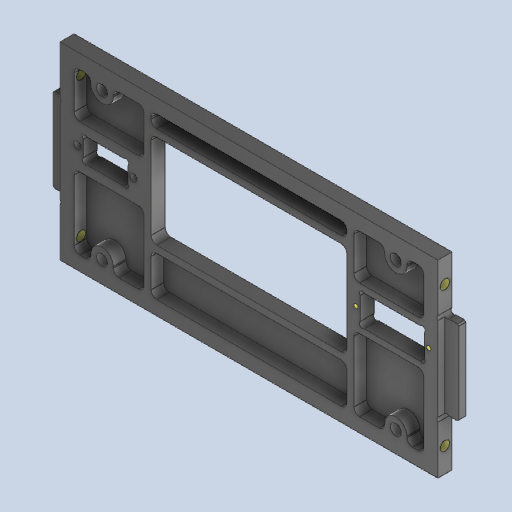
# Autodesk Inventor part: Cockpit_back_frame
Saved by Autodesk Inventor 2022.3 (Build 263350000, 350)
## iProperties
Part Number: Cockpit_back_frame
Material: アセタール樹脂、黒
Document SubType Name: Modeling
Designer: Masato Kubotera
Density: 1.425 g/cm^3
Appearance: 滑らか - 黒
Description: POM T5
Mass: 27.6157 g
Surface Area: 210.6 cm^2
Volume: 19.3794 cm^3
Author: Masato Kubotera
Autodesk Inventor part; units mm, degrees
ref_plane "XZ Plane" through (0, 0, 0) normal (0, 1, 0) x (-1, 0, 0)
derived "Cockpit_side_frame.ipt"
sketch "スケッチ2" plane through (0, 0, 0) normal (0, 1, 0) x (-1, 0, 0)
  line L0 (-23.5, -22.5) -> (-28.5, -27.5)
  line L1 (-28.5, -27.5) -> (-28.5, -91)
  line L2 (-28.5, -91) -> (-23.5, -96)
  line L3 (-23.5, -96) -> (34.25, -96)
  line L4 (36.25, -98) -> (36.25, -128.5)
  line L5 (36.25, -128.5) -> (46.25, -138.5)
  line L6 (46.25, -138.5) -> (86.5, -138.5)
  line L7 (91.5, -133.5) -> (91.5, -20)
  line L8 (91.5, -20) -> (89, -17.5)
  line L9 (89, -17.5) -> (83.25, -17.5)
  line L10 (83.25, -17.5) -> (83.25, -21.0151)
  line L11 (81.7651, -22.5) -> (76.8599, -22.5)
  line L12 (75.375, -21.0151) -> (75.375, -17.5)
  line L13 (75.375, -17.5) -> (60.375, -17.5)
  line L14 (60.375, -17.5) -> (60.375, -21.0151)
  line L15 (58.8901, -22.5) -> (-23.5, -22.5)
  line L16 (-25.25, -25) -> (-20.25, -25) construction
  line L17 (-20.25, -25) -> (-20.25, -93.5) construction
  line L18 (-20.25, -93.5) -> (-25.25, -93.5) construction
  line L19 (-25.25, -93.5) -> (-25.25, -25) construction
  line L20 (-26, -25) -> (-25.25, -25) construction
  line L21 (-25.25, -93.5) -> (-26, -93.5) construction
  line L22 (-26, -93.5) -> (-26, -25) construction
  line L23 (-20.25, -93.5) -> (83.25, -93.5) construction
  line L24 (-20.25, -88.5) -> (83.25, -88.5) construction
  line L25 (83.25, -22.5) -> (83.25, -90) construction
  line L26 (83.25, -90) -> (88.25, -90) construction
  line L27 (88.25, -90) -> (88.25, -22.5) construction
  line L28 (83.25, -88.5) -> (83.25, -93.5) construction
  line L29 (83.25, -91) -> (88.25, -91) construction
  line L30 (88.25, -91) -> (88.25, -136) construction
  line L31 (83.25, -91) -> (83.25, -136) construction
  line L32 (83.25, -136) -> (88.25, -136) construction
  line L33 (38.75, -131) -> (38.75, -93.5) construction
  line L34 (43.75, -93.5) -> (43.75, -131) construction
  line L35 (38.75, -131) -> (43.75, -131) construction
  line L36 (41.25, -131) -> (41.25, -93.5) construction
  line L37 (43.75, -131) -> (81.25, -131) construction
  line L38 (81.25, -131) -> (81.25, -136) construction
  line L39 (81.25, -136) -> (43.75, -136) construction
  line L40 (43.75, -133.5) -> (81.25, -133.5) construction
  line L41 (85.75, -91) -> (85.75, -136) construction
  circle A0 centre (85.75, -133.5) radius 2.975
  arc A1 (83.25, -131) -> (88.25, -131) centre (85.75, -133.5) ccw construction
  line L42 (83.25, -91) -> (-20.25, -91) construction
  line L43 (41.25, -112.25) -> (43.75, -112.25) construction
  line L44 (62.5, -131) -> (62.5, -133.5) construction
  line L45 (41.2, -116.8151) -> (41.2, -107.6849)
  line L46 (43.8, -108.3) -> (43.8, -116.2)
  line L47 (43.8, -118.3) -> (41.2, -106.2) construction
  line L48 (41.2, -118.3) -> (43.8, -106.2) construction
  line L49 (58.55, -130.95) -> (66.45, -130.95)
  line L50 (67.0651, -133.55) -> (57.9349, -133.55)
  line L51 (56.45, -130.95) -> (68.55, -133.55) construction
  line L52 (68.55, -130.95) -> (56.45, -133.55) construction
  line L53 (41.25, -106.25) -> (43.75, -106.25) construction
  line L54 (41.25, -118.25) -> (43.75, -118.25) construction
  arc A2 (42.6849, -106.2) -> (41.2, -107.6849) centre (41.9425, -106.9425) ccw
  arc A3 (43.8, -108.3) -> (43.8, -106.2) centre (43.8, -107.25) ccw
  arc A4 (41.2, -116.8151) -> (42.6849, -118.3) centre (41.9425, -117.5575) ccw
  arc A5 (43.8, -118.3) -> (43.8, -116.2) centre (43.8, -117.25) ccw
  line L55 (56.5, -133.5) -> (56.5, -131) construction
  line L56 (68.5, -131) -> (68.5, -133.5) construction
  arc A6 (56.45, -132.0651) -> (57.9349, -133.55) centre (57.1925, -132.8075) ccw
  arc A7 (58.55, -130.95) -> (56.45, -130.95) centre (57.5, -130.95) ccw
  arc A8 (67.0651, -133.55) -> (68.55, -132.0651) centre (67.8075, -132.8075) ccw
  arc A9 (68.55, -130.95) -> (66.45, -130.95) centre (67.5, -130.95) ccw
  line L57 (56.45, -132.0651) -> (56.45, -130.95)
  line L58 (68.55, -130.95) -> (68.55, -132.0651)
  line L59 (42.6849, -106.2) -> (43.8, -106.2)
  line L60 (43.8, -118.3) -> (42.6849, -118.3)
  circle A10 centre (48.75, -133.5) radius 1.6
  line L61 (88.25, -22.5) -> (88.25, -17.5) construction
  line L62 (89, -17.5) -> (89, -90) construction
  line L63 (89, -90) -> (88.25, -90) construction
  line L64 (-13.5, -82.5) -> (-13.5, -61)
  arc A11 (-13.5, -82.5) -> (-11.5, -84.5) centre (-11.5, -82.5) ccw
  line L65 (45.5, -84.5) -> (-11.5, -84.5)
  arc A12 (45.5, -84.5) -> (47.5, -82.5) centre (45.5, -82.5) ccw
  line L66 (47.5, -61) -> (47.5, -82.5)
  arc A13 (47.5, -61) -> (45.5, -59) centre (45.5, -61) ccw
  line L67 (-11.5, -59) -> (45.5, -59)
  arc A14 (-11.5, -59) -> (-13.5, -61) centre (-11.5, -61) ccw
  line L68 (31.5, -88.5) -> (31.5, -91) construction
  line L69 (85.75, -22.5) -> (85.75, -90) construction
  circle A15 centre (85.75, -31.25) radius 1.6
  circle A16 centre (85.75, -31.25) radius 3
  circle A17 centre (85.75, -81.25) radius 3
  circle A18 centre (85.75, -81.25) radius 1.6
  line L70 (88.25, -22.5) -> (83.25, -22.5) construction
  arc A19 (88.25, -91) -> (83.25, -91) centre (85.75, -133.5) ccw construction
  circle A20 centre (48.75, -133.5) radius 3
  circle A21 centre (41.25, -98.5) radius 1.6
  circle A22 centre (41.25, -98.5) radius 3
  line L71 (10.55, -88.5) -> (10.55, -91) construction
  line L72 (52.45, -88.5) -> (52.45, -91) construction
  line L73 (51.0151, -91.05) -> (11.9849, -91.05)
  line L74 (10.5, -89.5651) -> (10.5, -88.45)
  line L75 (12.6, -88.45) -> (50.4, -88.45)
  line L76 (52.5, -88.45) -> (52.5, -89.5651)
  line L77 (52.5, -91.05) -> (10.5, -88.45) construction
  line L78 (10.5, -91.05) -> (52.5, -88.45) construction
  arc A23 (12.6, -88.45) -> (10.5, -88.45) centre (11.55, -88.45) ccw
  arc A24 (10.5, -89.5651) -> (11.9849, -91.05) centre (11.2425, -90.3075) ccw
  arc A25 (51.0151, -91.05) -> (52.5, -89.5651) centre (51.7575, -90.3075) ccw
  arc A26 (52.5, -88.45) -> (50.4, -88.45) centre (51.45, -88.45) ccw
  line L79 (-20.25, -31) -> (83.25, -31) construction
  line L80 (83.25, -26) -> (-20.25, -26) construction
  line L81 (-20.25, -26) -> (-20.25, -31) construction
  line L82 (-20.25, -28.5) -> (83.25, -28.5) construction
  line L83 (31.5, -31) -> (31.5, -26) construction
  line L84 (11.9849, -31) -> (51.0151, -31)
  arc A27 (10.5, -29.5151) -> (11.9849, -31) centre (11.2425, -30.2575) ccw
  arc A28 (51.0151, -31) -> (52.5, -29.5151) centre (51.7575, -30.2575) ccw
  line L85 (10.55, -31) -> (10.55, -26) construction
  line L86 (52.45, -26) -> (52.45, -31) construction
  circle A29 centre (6.5, -28.5) radius 1.6
  circle A30 centre (6.5, -28.5) radius 3
  line L87 (-26, -59.25) -> (-25.25, -59.25) construction
  line L88 (-22.75, -25) -> (-22.75, -93.5) construction
  arc A31 (58.8901, -22.5) -> (60.375, -21.0151) centre (59.6325, -21.7575) ccw
  arc A32 (75.375, -21.0151) -> (76.8599, -22.5) centre (76.1175, -21.7575) ccw
  line L89 (56.4375, -22.5) -> (56.4375, -17.5) construction
  line L90 (79.3125, -22.5) -> (79.3125, -17.5) construction
  circle A33 centre (-22.75, -31.75) radius 1.6
  circle A34 centre (-22.75, -31.75) radius 3
  circle A35 centre (-22.75, -86.75) radius 1.6
  circle A36 centre (-22.75, -86.75) radius 3
  line L91 (60.375, -22.5) -> (75.375, -22.5)
  line L92 (52.5, -17.5) -> (52.5, -22.5) construction
  circle A37 centre (85.75, -98.5) radius 1.475
  circle A38 centre (85.75, -103.5) radius 1.475
  circle A39 centre (85.75, -108.5) radius 1.475
  line L93 (59.5, -88.5) -> (78.75, -88.5)
  line L94 (80.75, -90.5) -> (80.75, -126.5)
  line L95 (78.75, -128.5) -> (48.25, -128.5)
  line L96 (46.25, -126.5) -> (46.25, -110)
  arc A40 (46.25, -126.5) -> (48.25, -128.5) centre (48.25, -126.5) ccw
  arc A41 (78.75, -128.5) -> (80.75, -126.5) centre (78.75, -126.5) ccw
  arc A42 (80.75, -90.5) -> (78.75, -88.5) centre (78.75, -90.5) ccw
  arc A43 (36.25, -98) -> (34.25, -96) centre (34.25, -98) ccw
  circle A44 centre (-13.5, -55) radius 1.75
  circle A45 centre (-13.5, -55) radius 2
  line L97 (23.9, -43.85) -> (10.1, -43.85) construction
  line L98 (10.1, -43.85) -> (10.1, -34.65) construction
  line L99 (10.1, -34.65) -> (23.9, -34.65) construction
  line L100 (23.9, -34.65) -> (23.9, -43.85) construction
  line L101 (23.9, -43.85) -> (10.1, -34.65) construction
  line L102 (10.1, -43.85) -> (23.9, -34.65) construction
  line L103 (9.45, -33.95) -> (24.55, -33.95) construction
  line L104 (24.55, -33.95) -> (24.55, -44.55) construction
  line L105 (24.55, -44.55) -> (9.45, -44.55) construction
  line L106 (9.45, -44.55) -> (9.45, -33.95) construction
  line L107 (9.45, -33.95) -> (24.55, -44.55) construction
  line L108 (24.55, -33.95) -> (9.45, -44.55) construction
  line L109 (10.8849, -33.9) -> (23.1151, -33.9)
  line L110 (24.6, -35.3849) -> (24.6, -43.1151)
  line L111 (24.6, -44.6) -> (9.4, -33.9) construction
  line L112 (9.4, -44.6) -> (24.6, -33.9) construction
  line L113 (23.95, -43.9) -> (10.05, -34.6) construction
  line L114 (10.05, -43.9) -> (23.95, -34.6) construction
  arc A46 (10.8849, -33.9) -> (9.4, -35.3849) centre (10.1425, -34.6425) ccw
  arc A47 (11.5349, -34.6) -> (10.05, -36.0849) centre (10.7925, -35.3425) ccw
  line L115 (9.4, -39.25) -> (24.6, -39.25) construction
  line L116 (17, -33.9) -> (17, -44.6) construction
  arc A48 (24.6, -35.3849) -> (23.1151, -33.9) centre (23.8575, -34.6425) ccw
  arc A49 (23.95, -36.0849) -> (22.4651, -34.6) centre (23.2075, -35.3425) ccw
  arc A50 (10.05, -42.4151) -> (11.5349, -43.9) centre (10.7925, -43.1575) ccw
  arc A51 (9.4, -43.1151) -> (10.8849, -44.6) centre (10.1425, -43.8575) ccw
  arc A52 (22.4651, -43.9) -> (23.95, -42.4151) centre (23.2075, -43.1575) ccw
  arc A53 (23.1151, -44.6) -> (24.6, -43.1151) centre (23.8575, -43.8575) ccw
  line L117 (11.5349, -34.6) -> (22.4651, -34.6)
  line L118 (23.95, -36.0849) -> (23.95, -42.4151)
  line L119 (9.4, -43.1151) -> (9.4, -35.3849)
  line L120 (10.05, -42.4151) -> (10.05, -36.0849)
  line L121 (22.4651, -43.9) -> (11.5349, -43.9)
  line L122 (23.1151, -44.6) -> (10.8849, -44.6)
  line L123 (-13.5, -71.75) -> (47.5, -71.75) construction
  line L124 (85.75, -56.25) -> (88.25, -56.25) construction
  line L125 (85.7, -69.2) -> (85.7, -43.3)
  line L126 (88.3049, -71.3569) -> (85.7, -41.2) construction
  line L127 (85.7, -71.3) -> (88.3, -41.2) construction
  arc A54 (85.7, -41.2) -> (85.7, -43.3) centre (85.7, -42.25) ccw
  arc A55 (88.3, -42.6849) -> (86.8151, -41.2) centre (87.5575, -41.9425) ccw
  arc A56 (85.7, -69.2) -> (85.7, -71.3) centre (85.7, -70.25) ccw
  arc A57 (86.8151, -71.3) -> (88.3, -69.8151) centre (87.5575, -70.5575) ccw
  line L128 (85.75, -41.25) -> (88.25, -41.25) construction
  line L129 (85.75, -71.25) -> (88.25, -71.25) construction
  line L130 (88.3, -42.6849) -> (88.3, -69.8151)
  line L131 (88.3, -66.8652) -> (88.3, -69.8151)
  line L132 (86.8151, -71.3) -> (85.7, -71.3)
  line L133 (85.7, -41.2) -> (86.8151, -41.2)
  line L134 (86.5, -138.5) -> (91.5, -133.5)
  arc A58 (81.7651, -22.5) -> (83.25, -21.0151) centre (82.5075, -21.7575) ccw
  circle A59 centre (85.75, -93.5) radius 2
  circle A60 centre (85.75, -93.5) radius 4 construction
  arc A61 (-13.5, -49) -> (-11.5, -51) centre (-11.5, -49) ccw construction
  line L135 (45.5, -51) -> (-11.5, -51) construction
  arc A62 (45.5, -51) -> (47.5, -49) centre (45.5, -49) ccw construction
  line L136 (10.5, -29.5151) -> (10.5, -22.5)
  line L137 (52.5, -29.5151) -> (52.5, -22.5)
  line L138 (67.875, -17.5) -> (67.875, -22.5) construction
  line L139 (52.5, -17.5) -> (83.25, -17.5) construction
  line L140 (43.75, -131) -> (43.75, -136) construction
  line L141 (57.5, -22.5) -> (57.5, -103) construction
  line L142 (57.5, -103) -> (52.5, -108) construction
  line L143 (-23.5, -108) -> (52.5, -108) construction
  line L144 (57.5, -90.5) -> (57.5, -103)
  line L145 (57.5, -103) -> (52.5, -108)
  line L146 (52.5, -108) -> (48.25, -108)
  arc A63 (59.5, -88.5) -> (57.5, -90.5) centre (59.5, -90.5) ccw
  arc A64 (48.25, -108) -> (46.25, -110) centre (48.25, -110) ccw
  circle A65 centre (56.5, -28.5) radius 3
  circle A66 centre (56.5, -28.5) radius 1.6
  line L147 (-13.5, -49) -> (-13.5, -29.5)
  point P0 (0, 0)
  point P1 (-25.7227, -96)
  point P2 (-23.5, -22.5)
  point P3 (42.5, -112.25)
  point P4 (62.5, -132.25)
  point P5 (31.5, -89.75)
  point P6 (31.5, -28.5)
  point P7 (52.5, -22)
  point P8 (46.25, -108)
  point P9 (57.5, -88.5)
  point P10 (17, -39.25)
  point P11 (17, -39.25)
  point P12 (87, -56.25)
  point P13 (17, -51)
  point P14 (10.5, -31)
  point P15 (-13.5, -39.25)
  dimension "d2" = 88.25
  dimension "d10" = 2.5
  dimension "d11" = 5
  measures "d2" distance from line of L27 point (0, 0)
  measures "d10" distance of L129.start L129.end
  measures "d11" distance of L25.end L26.end
ref_plane "作業平面1" through (-88.25, 0, 0) normal (1, 0, 0) x (0, 1, 0)
sketch "スケッチ3" plane through (-88.25, 0, 0) normal (1, 0, 0) x (0, 1, 0)
  line L0 (-135, -22.5) -> (0, -22.5)
  line L1 (0, -22.5) -> (0, -39.7651)
  line L2 (0, -90) -> (-135, -90)
  line L3 (-135, -56.25) -> (0, -56.25) construction
  line L4 (-67.5, -22.5) -> (-67.5, -90) construction
  line L5 (1.4849, -41.25) -> (5, -41.25)
  line L6 (5, -41.25) -> (5, -71.25)
  line L7 (5, -71.25) -> (1.4849, -71.25)
  arc A0 (0, -39.7651) -> (1.4849, -41.25) centre (0.7425, -40.5075) ccw
  arc A1 (1.4849, -71.25) -> (0, -72.7349) centre (0.7425, -71.9925) ccw
  line L8 (0, -41.25) -> (0, -71.25)
  line L9 (0, -72.7349) -> (0, -90)
  line L10 (-135, -22.5) -> (-135, -39.7651)
  line L11 (-136.4849, -41.25) -> (-140, -41.25)
  line L12 (-140, -41.25) -> (-140, -71.25)
  line L13 (-140, -71.25) -> (-136.4849, -71.25)
  arc A2 (-136.4849, -41.25) -> (-135, -39.7651) centre (-135.7425, -40.5075) ccw
  arc A3 (-135, -72.7349) -> (-136.4849, -71.25) centre (-135.7425, -71.9925) ccw
  line L14 (-135, -41.25) -> (-135, -71.25)
  line L15 (-135, -72.7349) -> (-135, -90)
  line L16 (-100.5, -34.65) -> (-34.5, -34.65)
  line L17 (-32.5, -36.65) -> (-32.5, -66.15)
  line L18 (-34.5, -68.15) -> (-100.5, -68.15)
  line L19 (-102.5, -66.15) -> (-102.5, -36.65)
  arc A4 (-100.5, -34.65) -> (-102.5, -36.65) centre (-100.5, -36.65) ccw
  arc A5 (-102.5, -66.15) -> (-100.5, -68.15) centre (-100.5, -66.15) ccw
  arc A6 (-34.5, -68.15) -> (-32.5, -66.15) centre (-34.5, -66.15) ccw
  arc A7 (-32.5, -36.65) -> (-34.5, -34.65) centre (-34.5, -36.65) ccw
  line L20 (-111, -47.35) -> (-126.5, -47.35) construction
  line L21 (-126.5, -47.35) -> (-126.5, -55.45) construction
  line L22 (-126.5, -55.45) -> (-111, -55.45) construction
  line L23 (-111, -55.45) -> (-111, -47.35) construction
  line L24 (-111, -47.35) -> (-126.5, -55.45) construction
  line L25 (-126.5, -47.35) -> (-111, -55.45) construction
  line L26 (-126.75, -55.7) -> (-110.75, -55.7)
  line L27 (-110.75, -55.7) -> (-110.75, -47.1)
  line L28 (-110.75, -47.1) -> (-126.75, -47.1)
  line L29 (-126.75, -47.1) -> (-126.75, -55.7)
  line L30 (-126.75, -55.7) -> (-110.75, -47.1) construction
  line L31 (-110.75, -55.7) -> (-126.75, -47.1) construction
  line L32 (-108.75, -51.4) -> (-128.75, -51.4) construction
  line L33 (-118.75, -47.1) -> (-118.75, -55.7) construction
  circle A8 centre (-108.75, -51.4) radius 1.35
  circle A9 centre (-108.75, -51.4) radius 2.25 construction
  circle A10 centre (-128.75, -51.4) radius 1.35
  line L34 (-27.5, -56.65) -> (-5, -56.65) construction
  line L35 (-27.75, -56.9) -> (-4.75, -56.9)
  line L36 (-27.5, -46.15) -> (-27.5, -56.65) construction
  line L37 (-5, -56.65) -> (-5, -46.15) construction
  line L38 (-5, -46.15) -> (-27.5, -46.15) construction
  line L39 (-27.5, -46.15) -> (-5, -56.65) construction
  line L40 (-27.5, -56.65) -> (-5, -46.15) construction
  line L41 (-16.25, -46.15) -> (-16.25, -56.65) construction
  line L42 (-27.75, -45.9) -> (-27.75, -56.9)
  line L43 (-4.75, -56.9) -> (-4.75, -45.9)
  line L44 (-4.75, -45.9) -> (-27.75, -45.9)
  line L45 (-27.75, -45.9) -> (-4.75, -56.9) construction
  line L46 (-27.75, -56.9) -> (-4.75, -45.9) construction
  circle A11 centre (-3.25, -51.4) radius 0.8
  arc A12 (-4.75, -47.3849) -> (-6.2349, -45.9) centre (-5.4925, -46.6425) ccw
  arc A13 (-6.2349, -56.9) -> (-4.75, -55.4151) centre (-5.4925, -56.1575) ccw
  line L47 (-29.25, -51.4) -> (-3.25, -51.4) construction
  arc A14 (-27.75, -55.4151) -> (-26.2651, -56.9) centre (-27.0075, -56.1575) ccw
  circle A15 centre (-29.25, -51.4) radius 0.8
  arc A16 (-26.2651, -45.9) -> (-27.75, -47.3849) centre (-27.0075, -46.6425) ccw
  arc A17 (-110.75, -48.5849) -> (-112.2349, -47.1) centre (-111.4925, -47.8425) ccw
  arc A18 (-125.2651, -47.1) -> (-126.75, -48.5849) centre (-126.0075, -47.8425) ccw
  arc A19 (-126.75, -54.2151) -> (-125.2651, -55.7) centre (-126.0075, -54.9575) ccw
  arc A20 (-112.2349, -55.7) -> (-110.75, -54.2151) centre (-111.4925, -54.9575) ccw
  line L48 (-130, -29.5) -> (-130, -41.65)
  line L49 (-128, -43.65) -> (-107, -43.65)
  line L50 (-128, -27.5) -> (-126, -27.5)
  line L51 (-105, -29.5) -> (-105, -41.65)
  line L52 (-28, -27.5) -> (-21, -27.5)
  line L53 (-5, -29.5) -> (-5, -41.65)
  line L54 (-7, -43.65) -> (-28, -43.65)
  line L55 (-30, -41.65) -> (-30, -29.5)
  line L56 (-100.5, -27.5) -> (-34.5, -27.5)
  line L57 (-32.5, -29.5) -> (-32.5, -30.15)
  line L58 (-34.5, -32.15) -> (-100.5, -32.15)
  line L59 (-102.5, -30.15) -> (-102.5, -29.5)
  line L60 (-128, -59.15) -> (-107, -59.15)
  line L61 (-7, -59.15) -> (-28, -59.15)
  line L62 (-34.5, -70.65) -> (-100.5, -70.65)
  line L63 (-128, -85) -> (-126, -85)
  line L64 (-28, -85) -> (-21, -85)
  line L65 (-100.5, -85) -> (-34.5, -85)
  line L66 (-130, -61.15) -> (-130, -83)
  line L67 (-105, -61.15) -> (-105, -83)
  line L68 (-102.5, -83) -> (-102.5, -72.65)
  line L69 (-32.5, -72.65) -> (-32.5, -83)
  line L70 (-30, -83) -> (-30, -61.15)
  line L71 (-5, -61.15) -> (-5, -83)
  arc A21 (-128, -27.5) -> (-130, -29.5) centre (-128, -29.5) ccw
  arc A22 (-130, -41.65) -> (-128, -43.65) centre (-128, -41.65) ccw
  arc A23 (-107, -43.65) -> (-105, -41.65) centre (-107, -41.65) ccw
  arc A24 (-105, -29.5) -> (-107, -27.5) centre (-107, -29.5) ccw
  arc A25 (-100.5, -27.5) -> (-102.5, -29.5) centre (-100.5, -29.5) ccw
  arc A26 (-102.5, -30.15) -> (-100.5, -32.15) centre (-100.5, -30.15) ccw
  arc A27 (-34.5, -32.15) -> (-32.5, -30.15) centre (-34.5, -30.15) ccw
  arc A28 (-32.5, -29.5) -> (-34.5, -27.5) centre (-34.5, -29.5) ccw
  arc A29 (-28, -27.5) -> (-30, -29.5) centre (-28, -29.5) ccw
  arc A30 (-5, -29.5) -> (-7, -27.5) centre (-7, -29.5) ccw
  arc A31 (-7, -43.65) -> (-5, -41.65) centre (-7, -41.65) ccw
  arc A32 (-30, -41.65) -> (-28, -43.65) centre (-28, -41.65) ccw
  arc A33 (-28, -59.15) -> (-30, -61.15) centre (-28, -61.15) ccw
  arc A34 (-30, -83) -> (-28, -85) centre (-28, -83) ccw
  arc A35 (-7, -85) -> (-5, -83) centre (-7, -83) ccw
  arc A36 (-5, -61.15) -> (-7, -59.15) centre (-7, -61.15) ccw
  arc A37 (-34.5, -85) -> (-32.5, -83) centre (-34.5, -83) ccw
  arc A38 (-32.5, -72.65) -> (-34.5, -70.65) centre (-34.5, -72.65) ccw
  arc A39 (-102.5, -83) -> (-100.5, -85) centre (-100.5, -83) ccw
  arc A40 (-100.5, -70.65) -> (-102.5, -72.65) centre (-100.5, -72.65) ccw
  arc A41 (-107, -85) -> (-105, -83) centre (-107, -83) ccw
  arc A42 (-105, -61.15) -> (-107, -59.15) centre (-107, -61.15) ccw
  arc A43 (-128, -59.15) -> (-130, -61.15) centre (-128, -61.15) ccw
  arc A44 (-130, -83) -> (-128, -85) centre (-128, -83) ccw
  circle A45 centre (-15, -30) radius 2
  arc A46 (-11.4799, -32.1) -> (-11.4799, -27.9) centre (-7.5, -30) ccw construction
  line L72 (-7.5, -30) -> (-15, -30) construction
  arc A47 (-15, -27.9) -> (-15, -32.1) centre (-15, -30) ccw construction
  line L73 (-15, -27.9) -> (-11.4799, -27.9) construction
  line L74 (-15, -32.1) -> (-11.4799, -32.1) construction
  circle A48 centre (-15, -30) radius 3 construction
  line L75 (-11, -30) -> (-11, -29.5)
  line L76 (-19, -30) -> (-19, -29.5)
  arc A49 (-19, -30) -> (-11, -30) centre (-15, -30) ccw
  line L77 (-9, -27.5) -> (-7, -27.5)
  arc A50 (-120, -32.1) -> (-120, -27.9) centre (-120, -30) ccw construction
  circle A51 centre (-120, -30) radius 2
  circle A52 centre (-120, -30) radius 3 construction
  line L78 (-120, -32.1) -> (-123.5201, -32.1) construction
  line L79 (-120, -27.9) -> (-123.5201, -27.9) construction
  arc A53 (-123.5201, -27.9) -> (-123.5201, -32.1) centre (-127.5, -30) ccw construction
  arc A54 (-124, -30) -> (-116, -30) centre (-120, -30) ccw
  line L80 (-124, -30) -> (-124, -29.5)
  line L81 (-116, -30) -> (-116, -29.5)
  line L82 (-114, -27.5) -> (-107, -27.5)
  arc A55 (-15, -80.4) -> (-15, -84.6) centre (-15, -82.5) ccw construction
  circle A56 centre (-15, -82.5) radius 2
  circle A57 centre (-15, -82.5) radius 3 construction
  line L83 (-15, -80.4) -> (-11.4799, -80.4) construction
  line L84 (-15, -84.6) -> (-11.4799, -84.6) construction
  line L85 (-7.5, -82.5) -> (-15, -82.5) construction
  arc A58 (-11.4799, -84.6) -> (-11.4799, -80.4) centre (-7.5, -82.5) ccw construction
  arc A59 (-11, -82.5) -> (-19, -82.5) centre (-15, -82.5) ccw
  line L86 (-19, -82.5) -> (-19, -83)
  line L87 (-116, -82.5) -> (-116, -83)
  arc A60 (-116, -82.5) -> (-124, -82.5) centre (-120, -82.5) ccw
  circle A61 centre (-120, -82.5) radius 3 construction
  line L88 (-120, -84.6) -> (-123.5201, -84.6) construction
  arc A62 (-120, -84.6) -> (-120, -80.4) centre (-120, -82.5) ccw construction
  circle A63 centre (-120, -82.5) radius 2
  arc A64 (-123.5201, -80.4) -> (-123.5201, -84.6) centre (-127.5, -82.5) ccw construction
  line L89 (-124, -82.5) -> (-124, -83)
  line L90 (-11, -82.5) -> (-11, -83)
  line L91 (-9, -85) -> (-7, -85)
  line L92 (-120, -80.4) -> (-123.5201, -80.4) construction
  line L93 (-114, -85) -> (-107, -85)
  arc A65 (-126, -85) -> (-124, -83) centre (-126, -83) ccw
  arc A66 (-116, -83) -> (-114, -85) centre (-114, -83) ccw
  arc A67 (-124, -29.5) -> (-126, -27.5) centre (-126, -29.5) ccw
  arc A68 (-114, -27.5) -> (-116, -29.5) centre (-114, -29.5) ccw
  arc A69 (-19, -29.5) -> (-21, -27.5) centre (-21, -29.5) ccw
  arc A70 (-9, -27.5) -> (-11, -29.5) centre (-9, -29.5) ccw
  arc A71 (-21, -85) -> (-19, -83) centre (-21, -83) ccw
  arc A72 (-11, -83) -> (-9, -85) centre (-9, -83) ccw
  point P0 (0, 0)
  point P1 (-135, -71.25)
  point P2 (-67.5, -34.65)
  point P3 (-118.75, -51.4)
  point P4 (-118.75, -51.4)
  point P5 (-16.25, -51.4)
  point P6 (-16.25, -51.4)
  point P7 (-126.75, -48.5849)
  point P8 (-125.2651, -47.1)
  point P9 (-110.75, -54.2151)
  point P10 (-126.75, -54.2151)
  point P11 (-26.2651, -56.9)
  point P12 (-27.75, -55.4151)
  point P13 (-6.2349, -45.9)
  point P14 (-4.75, -47.3849)
  point P15 (-4.75, -55.4151)
  point P16 (-6.2349, -56.9)
  point P17 (-130, -27.5)
  point P18 (-130, -43.65)
  point P19 (-105, -27.5)
  point P20 (-105, -43.65)
  point P21 (-30, -27.5)
  point P22 (-5, -43.65)
  point P23 (-5, -27.5)
  point P24 (-30, -43.65)
  point P25 (-102.5, -27.5)
  point P26 (-32.5, -32.15)
  point P27 (-32.5, -27.5)
  point P28 (-102.5, -32.15)
  point P29 (-130, -59.15)
  point P30 (-105, -59.15)
  point P31 (-5, -59.15)
  point P32 (-30, -59.15)
  point P33 (-32.5, -70.65)
  point P34 (-102.5, -70.65)
  point P35 (-130, -85)
  point P36 (-105, -85)
  point P37 (-30, -85)
  point P38 (-5, -85)
  point P39 (-102.5, -85)
  point P40 (-32.5, -85)
  point P41 (-102.5, -51.4)
  point P42 (-11, -27.5)
  point P43 (-19, -27.5)
  point P44 (-3, -30)
  point P45 (-116, -27.5)
  point P46 (-124, -27.5)
  point P47 (-19, -85)
  point P48 (-116, -85)
  point P49 (-124, -85)
  point P50 (-11, -85)
  point P51 (-118.75, -43.65)
  point P52 (-118.75, -51.4)
  point P53 (-16.25, -51.4)
  dimension "d3" = 1.05
  dimension "d4" = 135
  dimension "d5" = 5
  dimension "d20" = 2
  dimension "d22" = 70
  dimension "d25" = 15.5
  dimension "d26" = 8.1
  dimension "d28" = 0.25
  dimension "d29" = 20
  dimension "d30" = 2.7
  dimension "d31" = 4.5
  dimension "d33" = 10.5
  dimension "d34" = 22.5
  dimension "d35" = 26
  dimension "d36" = 1.6
  dimension "d37" = 1.05
  dimension "d38" = 23
  dimension "d39" = 11
  dimension "d41" = 1.05
  dimension "d49" = 5
  dimension "d50" = 5
  dimension "d51" = 2.5
  dimension "d53" = 2.5
  dimension "d54" = 2.5
  dimension "d55" = 2
  dimension "d58" = 0.25
  dimension "d59" = 8.6
  dimension "d60" = 16
  dimension "d65" = 33.5
  dimension "d66" = 4
  dimension "d67" = 9
  dimension "d68" = 4.2
  dimension "d69" = 6
  dimension "d70" = 4
  dimension "d71" = 3
  dimension "d72" = 3
  dimension "d74" = 32.5
  dimension "d75" = 16.25
  dimension "d76" = 16.25
  dimension "d77" = 32.5
  dimension "d78" = 28.9
  constraints: 186 end point, 126 point on circle, 86 tangent, 85 point on line, 84 symmetric about line, 73 centre point, 34 equal radius, 24 midpoint, 24 parallel, 19 perpendicular, 17 coincident, 12 horizontal, 6 collinear, 1 vertical, 33 other
  measures "d3" radius of A0
  measures "d4" distance of L0.start L0.end
  measures "d5" distance of L8.start L5.end
  measures "d20" radius of A4
  measures "d22" distance between parallel lines of L17 L19
  measures "d25" distance of L23.start L21.end
  measures "d26" distance of L21.end L21.start
  measures "d28" horizontal distance of L28.start L20.start
  measures "d29" distance of L32.start L32.end
  measures "d30" diameter of A8
  measures "d31" diameter of A9
  measures "d33" distance of L38.start L34.end
  measures "d34" distance of L34.end L34.start
  measures "d35" distance of L47.start L47.end
  measures "d36" diameter of A15
  measures "d37" radius of A16
  measures "d38" distance of L44.start L44.end
  measures "d39" distance of L44.end L35.start
  measures "d41" radius of A17
  measures "d49" distance between parallel lines of L0 L56
  measures "d50" distance between parallel lines of L10 L48
  measures "d51" distance between parallel lines of L51 L59
  measures "d53" distance between parallel lines of L38 L54
  measures "d54" distance between parallel lines of L16 L58
  measures "d55" radius of A21
  measures "d58" distance between parallel lines of L23 L27
  measures "d59" distance of L28.end L30.start
  measures "d60" distance of L28.start L28.end
  measures "d65" distance between parallel lines of L18 L16
  measures "d66" diameter of A45
  measures "d67" diameter of A46
  measures "d68" diameter of A47
  measures "d69" diameter of A48
  measures "d70" radius of A49
  measures "d71" distance edge to line of A46 L0
  measures "d72" distance from line of point (-3, -30) L1
  measures "d74" horizontal distance of L0.start L19.end
  measures "d75" horizontal distance of L0.start point (-118.75, -51.4)
  measures "d76" horizontal distance of point (-16.25, -51.4) point (0, -22.5)
  measures "d77" horizontal distance of L17.start L0.end
  measures "d78" vertical distance of L0.start point (-102.5, -51.4)
extrude "押し出し1" add sketch "スケッチ3" along normal blind 5 contours L0 L1 A0 L8 A1 L9 L2 L15 A3 L14 A2 L10
extrude "押し出し2" add sketch "スケッチ3" along normal blind 2.5 contours L14 A3 L13 L12 L11 A2 | A0 L5 L6 L7 A1 L8
hole "穴1" at (-85.75, 0, -81.25) at (-85.75, 0, -31.25) direction (0, -1, 0) diameter 3.4587 depth 10 thread size "M4x0.5" class "6H" standard "ISO Metric profile"
ref_plane "作業平面2" through (-88.25, -67.5, -22.5) normal (0, 1, 0) x (1, 0, 0)
mirror "ミラー1" about plane through (-88.25, -67.5, -22.5) normal (0, 1, 0) of "穴1"
extrude "押し出し3" add sketch "スケッチ3" along normal blind 0.5 contours A21 L50 A67 L80 A54 L81 A68 L82 A24 L51 A23 L49 A22 L48 | L52 A69 L76 A49 L75 A70 L77 A30 L53 A31 L54 A32 L55 A29 | L56 A28 L57 A27 L58 A26 L59 A25 | L60 A42 L67 A41 L93 A66 L87 A60 L89 A65 L63 A44 L66 A43 | A36 L71 A35 L91 A72 L90 A59 L86 A71 L64 A34 L70 A33 L61 | A38 L69 A37 L65 A39 L68 A40 L62
chamfer "面取り1" distance 0.5 angle 45 4 edges at (-87, -140, -71.25) (-87, -140, -41.25) (-87, 5, -71.25) (-87, 5, -41.25)
equation "\"d41\" = d42"
equation "\"d6\" = d11"
equation "\"d8\" = d10"
equation "\"d1\" = -d2"
equation "\"d42\" = 1.05"
